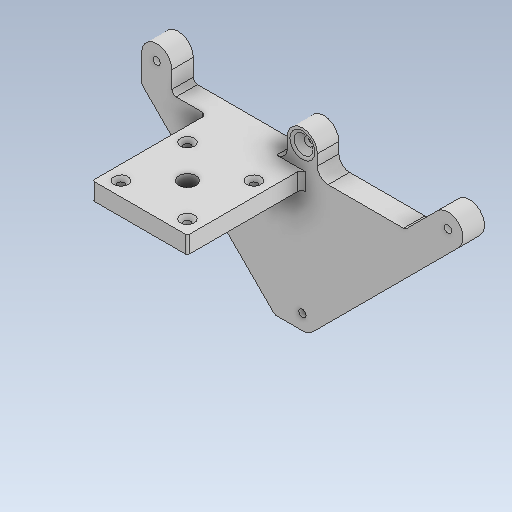
# Autodesk Inventor part: FourWireWinderBracket
Saved by Autodesk Inventor 2020.2 (Build 242310000, 310)
## iProperties
Created: 2020-03-15
Part Number: FourWireWinderBracket
Material: Generic
Document SubType Name: Modeling
Designer: elmar
Density: 1 g/cm^3
Appearance: Default
Author: elmar
Autodesk Inventor part; units mm, degrees
ref_plane "YZ Plane" through (0, 0, 0) normal (1, 0, 0) x (0, 1, 0)
ref_plane "XZ Plane" through (0, 0, 0) normal (0, 1, 0) x (-1, 0, 0)
ref_plane "XY Plane" through (0, 0, 0) normal (0, 0, 1) x (1, 0, 0)
sketch "Sketch1" plane through (0, 0, 0) normal (0, 0, 1) x (1, 0, 0)
  line L0 (-67.9674, 0) -> (0, 67.9674)
  line L1 (0, 67.9674) -> (67.9674, 0)
  line L2 (67.9674, 0) -> (0, -67.9674)
  line L3 (0, -67.9674) -> (-67.9674, 0)
  line L4 (-105, 0) -> (105, 0) projected
  line L5 (-75, 7.0326) -> (75, 7.0326)
  line L6 (75, 7.0326) -> (75, -75)
  line L7 (75, -75) -> (-75, -75)
  line L8 (-75, -75) -> (-75, 7.0326)
  line L9 (0, -103.5935) -> (0, 96.5608) projected
  line L10 (-60.9347, 7.0326) -> (60.9347, 7.0326)
  line L11 (60.9347, 7.0326) -> (60.9347, -10)
  line L12 (60.9347, -10) -> (-60.9347, -10)
  line L13 (-60.9347, -10) -> (-60.9347, 7.0326)
  circle A0 centre (67.9674, 0) radius 7.0326
  circle A1 centre (-67.9674, 0) radius 7.0326
  line L14 (-62.9945, 4.9728) -> (-48.0217, -10)
  line L15 (48.0217, -10) -> (62.9945, 4.9728)
  circle A2 centre (0, -67.9674) radius 7.0326
  line L16 (-72.9402, -4.9728) -> (-4.9728, -72.9402)
  line L17 (72.9402, -4.9728) -> (4.9728, -72.9402)
  line L18 (-75, -12.8587) -> (-12.8587, -75)
  point P0 (0, 0)
  point P1 (0, 0)
  point P2 (0, -75)
  point P3 (0, -10)
  point P4 (-60.9347, 0)
  point P5 (-75, 0)
  point P6 (0, -75)
  dimension "d55" = 3
  dimension "d0" = 67.9674
  dimension "d1" = 150
  dimension "d2" = 7.0326
  dimension "d3" = 7.0326
  dimension "d5" = 10
  dimension "d19" = 7.0326
  dimension "d64" = 96.1204
  constraints: 34 end point, 10 tangent, 8 point on line, 6 parallel, 6 point on circle, 4 coincident, 4 perpendicular, 3 centre point, 2 horizontal, 2 midpoint, 9 other
  measures "d0" distance of L0.start point (0, 0)
  measures "d1" distance of L6.end L7.end
  measures "d2" distance from line of L6 L1.end
  measures "d3" distance from line of L7 L2.end
  measures "d5" distance between parallel lines of L12 L4
  measures "d19" distance between parallel lines of L18 L16
  measures "d64" distance of L2.end L0.start
extrude "Extrusion1" add sketch "Sketch1" along normal blind 10 contours L4 A1 L0 | L4 A1 L3 | L0 A1 L4 | L3 A1 L4 | A1 L13 L3 | L3 L13 L12 A2 L16 A1 | A1 L16 A2 L7 L18 L8 | L12 L9 A2 L3 | A2 L3 L9 | A2 L9 L3 | L9 L2 A2 | L15 L11 L4 | L4 L11 L2 L12 L15 | L12 L2 A2 L9 | A0 L4 L1 | L1 L4 A0 | A0 L11 L15 | L9 A2 L2 | A2 L2 L12 L11 A0 L17 | A0 L2 L11 | L4 L2 A0 | L4 A0 L2 | L11 L12 L2
hole "Hole1" at (-67.9674, 0, 0) at (67.9674, 0, 0) at (0, -67.9674, 0) direction (0, 0, 1) diameter 3.4 end through all clearance for "Flat Head Machine Screw" size "M3" standard "Ansi Metric M Profile"
sketch "Sketch2" plane through (-48.0184, -10, 0) normal (0, 1, 0) x (1, 0, 0)
  circle A0 centre (25.5184, -41.15) radius 22.5
  line L0 (48.0184, 12.73) -> (48.0184, -76.38) projected
  line L1 (41.0184, -25.65) -> (41.0184, -56.65)
  line L2 (41.0184, -56.65) -> (10.0184, -56.65)
  line L3 (10.0184, -56.65) -> (10.0184, -25.65)
  line L4 (10.0184, -25.65) -> (41.0184, -25.65)
  line L5 (46.6684, -62.3) -> (4.3684, -62.3)
  line L6 (4.3684, -62.3) -> (4.3684, -20)
  line L7 (4.3684, -20) -> (46.6684, -20)
  line L8 (46.6684, -20) -> (46.6684, -62.3)
  line L9 (96.0401, -10) -> (-12.9164, -10) projected
  line L10 (3.3684, -63.3) -> (47.6684, -63.3)
  line L11 (47.6684, -63.3) -> (47.6684, -10)
  line L12 (47.6684, -10) -> (3.3684, -10)
  line L13 (3.3684, -10) -> (3.3684, -63.3)
  point P0 (48.0184, 0)
  point P1 (3.3684, -10)
  dimension "d15" = 45
  dimension "d16" = 31
  dimension "d17" = 42.3
  dimension "d18" = 10
  dimension "d21" = 1
  dimension "d22" = 1
  dimension "d23" = 1
  constraints: 24 end point, 2 coincident, 2 parallel, 2 vertical, 1 centre point, 1 horizontal, 1 perpendicular, 1 point on line, 1 tangent, 18 other
  measures "d15" diameter of A0
  measures "d16" distance of L1.end L2.end
  measures "d17" distance of L7.end L5.start
  measures "d18" distance between parallel lines of L9 L7
  measures "d21" distance between parallel lines of L8 L11
  measures "d22" distance between parallel lines of L5 L10
  measures "d23" distance between parallel lines of L6 L13
fillet "Fillet1" radius 2 4 edges at (-75, -12.8587, 5) (-12.8587, -75, 5) (48.0217, -10, 5) (-60.9347, -10, 5)
extrude "Extrusion2" add sketch "Sketch2" against normal blind 8 contours L11 A0 L8 | A0 L8 L7 L6 L13 L9 L11 | L11 L10 A0 L5 L8 | L8 A0 L5 L6 L7 | A0 L7 L8 | L8 L5 A0 | L7 A0 | A0 L10 L5 | A0 L6 L7 | A0 L6 L13 | L5 L6 A0 | A0 L10 L13 L6 L5 | L1 L2 L3 L4
hole "Hole2" at (-7, -10, 25.65) at (-7, -10, 56.65) at (-38, -10, 56.65) at (-38, -10, 25.65) direction (0, -1, 0) diameter 3.2 end through all countersink diameter 6.5 countersink angle 90 clearance for "Flat Head Machine Screw" size "M3" standard "Ansi Metric M Profile"
sketch "Sketch3" plane through (-48.0184, -18, 0) normal (0, -1, 0) x (1, 0, 0)
  circle A0 centre (25.5184, 41.15) radius 11.5
  point P0 (48.0184, 0)
  dimension "d40" = 23
  constraints: 1 centre point, 1 coincident
  measures "d40" diameter of A0
hole "Hole3" at (-22.5, -10, 41.15) direction (0, -1, 0) diameter 8 end through all
extrude "Extrusion3" cut sketch "Sketch3" against normal blind 2.2
fillet "Fillet2" radius 1 2 edges at (-44.65, -14, 63.3) (-0.35, -14, 63.3)
fillet "Fillet3" radius 2 2 edges at (-44.65, -14, 10) (-0.35, -14, 10)
sketch "Sketch4" plane through (0, 0, 0) normal (0, 0, -1) x (-1, 0, 0)
  circle A0 centre (0, 0) radius 7
  line L0 (-7, 0) -> (-7, -10)
  line L1 (-47.1933, -10) -> (-1.65, -10) projected
  line L2 (7, 0) -> (7, -10)
  line L3 (43.65, -10) -> (1.35, -10) projected
  line L4 (-47.1933, -10) -> (58.9347, -10) projected
  dimension "d45" = 14
  constraints: 4 end point, 2 point on circle, 2 point on line, 2 tangent, 1 centre point, 1 coincident, 1 parallel, 1 vertical
  measures "d45" diameter of A0
extrude "Extrusion4" add sketch "Sketch4" against normal up to surface (10 mm away)
hole "Hole4" at (0, 0, 0) direction (0, 0, 1) diameter 3 end through all countersink diameter 10 countersink angle 90
sketch "Sketch5" plane through (0, 0, 10) normal (0, 0, 1) x (1, 0, 0)
  point P0 (0, 0)
hole "Hole5" at (0, 0, 10) direction (0, 0, -1) diameter 3 end through all countersink diameter 10 countersink angle 90
fillet "Fillet4" radius 2 5 edges at (0, -1.5, 3.5) (-1.5, 0, 6.5) (1.5, 0, 6.5) (0, 5, 10) (0, -5, 0)
fillet "Fillet5" radius 5 2 edges at (7, -10, 5) (-7, -10, 5)
equation "\"d0\" = SupportHoleDistance"
equation "\"d1\" = SideLength"
equation "\"d3\" = d2"
equation "\"d19\" = d2"
equation "\"d6\" = d5"
equation "\"SideLength\" = 150"
equation "\"SupportHoleDistance\" = 67.967358"
body "Solid1"
